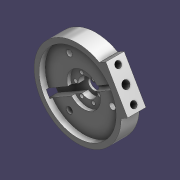
# Autodesk Inventor part: AA046
Saved by Autodesk Inventor 2017 SP1 (Build 210196100, 196)
## iProperties
Created: 2018-01-29
Part Number: AA046
Material: ABS Plastic
Document SubType Name: Modeling
Designer: Zach
Density: 1.06 g/cm^3
Appearance: CR White
Author: Zach
Autodesk Inventor part; units mm, degrees
ref_plane "YZ Plane" through (0, 0, 0) normal (1, 0, 0) x (0, 1, 0)
ref_plane "XZ Plane" through (0, 0, 0) normal (0, 1, 0) x (-1, 0, 0)
ref_plane "XY Plane" through (0, 0, 0) normal (0, 0, 1) x (1, 0, 0)
sketch "Sketch1" plane through (0, 0, 0) normal (0, 0, 1) x (1, 0, 0)
  circle A0 centre (0, 0) radius 35
  circle A1 centre (0, 0) radius 4.5
  dimension "d0" = 70
  dimension "d1" = 9
  constraints: 2 centre point, 2 coincident
  measures "d0" diameter of A0
  measures "d1" diameter of A1
extrude "Extrusion1" add sketch "Sketch1" along normal blind 14.75
sketch "Sketch2" plane through (0, 0, 14.75) normal (0, 0, 1) x (1, 0, 0)
  circle A0 centre (0, 0) radius 13.5
  dimension "d4" = 27
  constraints: 1 centre point, 1 coincident
  measures "d4" diameter of A0
extrude "Extrusion2" cut sketch "Sketch2" against normal blind 8
sketch "Sketch3" plane through (0, 0, 6.75) normal (0, 0, 1) x (1, 0, 0)
  circle A0 centre (0, 0) radius 7.5
  dimension "d7" = 15
  constraints: 1 centre point, 1 coincident
  measures "d7" diameter of A0
extrude "Extrusion3" cut sketch "Sketch3" against normal blind 5
sketch "Sketch4" plane through (0, 0, 6.75) normal (0, 0, 1) x (1, 0, 0)
  circle A0 centre (9.525, 0) radius 1.5
  circle A1 centre (4.7625, 8.2489) radius 1.5
  circle A2 centre (-4.7625, 8.2489) radius 1.5
  circle A3 centre (-9.525, 0) radius 1.5
  circle A4 centre (-4.7625, -8.2489) radius 1.5
  circle A5 centre (4.7625, -8.2489) radius 1.5
  point P0 (0, 0)
  dimension "d10" = 3
  dimension "d11" = 9.525
  dimension "d14" = 360
  constraints: 6 centre point, 1 horizontal alignment, 13 other
  measures "d10" diameter of A0
  measures "d11" distance of A0.centre point (0, 0)
extrude "Extrusion4" cut sketch "Sketch4" against normal through all
sketch "Sketch5" plane through (0, 0, 14.75) normal (0, 0, 1) x (1, 0, 0)
  circle A0 centre (23, 0) radius 2.5
  circle A1 centre (-11.5, 19.9186) radius 2.5
  circle A2 centre (-11.5, -19.9186) radius 2.5
  point P0 (0, 0)
  dimension "d18" = 5
  dimension "d19" = 23
  dimension "d22" = 360
  constraints: 3 centre point, 1 horizontal alignment, 7 other
  measures "d18" diameter of A0
  measures "d19" distance of A0.centre point (0, 0)
extrude "Extrusion5" cut sketch "Sketch5" against normal through all
sketch "Sketch6" plane through (0, 0, 14.75) normal (0, 0, 1) x (1, 0, 0)
  circle A0 centre (23, 0) radius 2.5 projected
  circle A1 centre (23, 0) radius 6.5
  circle A2 centre (11.5, 19.9186) radius 6.5
  circle A3 centre (-11.5, 19.9186) radius 6.5
  circle A4 centre (-23, 0) radius 6.5
  circle A5 centre (-11.5, -19.9186) radius 6.5
  circle A6 centre (11.5, -19.9186) radius 6.5
  point P0 (0, 0)
  dimension "d26" = 13
  dimension "d29" = 360
  constraints: 6 centre point, 1 coincident, 13 other
  measures "d26" diameter of A1
extrude "Extrusion6" cut sketch "Sketch6" against normal blind 5 contours A0 | A1 | A3 | A5
sketch "Sketch7" plane through (0, 0, 14.75) normal (0, 0, 1) x (1, 0, 0)
  line L0 (17.5, 30.3109) -> (22.6962, 33.3109)
  line L1 (22.6962, 33.3109) -> (40.1962, 3)
  line L2 (40.1962, 3) -> (35, 0)
  line L3 (35, 0) -> (17.5, 30.3109)
  circle A0 centre (0, 0) radius 35 construction
  line L4 (0, 0) -> (26.25, 15.1554)
  circle A1 centre (23, 0) radius 2.5 construction
  line L5 (0, 0) -> (23, 0)
  dimension "d33" = 6
  dimension "d34" = 35
  dimension "d43" = 30
  constraints: 12 end point, 2 parallel, 2 point on circle, 1 horizontal, 1 midpoint, 1 perpendicular
  measures "d33" distance of L0.start L0.end
  measures "d34" distance of L0.end L1.end
  measures "d43" angle of L5 L4
extrude "Extrusion7" add sketch "Sketch7" against normal blind 14.75
sketch "Sketch8" plane through (40.1962, 3, 14.75) normal (0.8660254, 0.5, 0) x (0, 0, -1)
  circle A0 centre (7.375, 30) radius 2.5
  circle A1 centre (7.375, 5) radius 2.5
  line L0 (7.375, 30) -> (7.375, 5) construction
  line L1 (14.75, 35) -> (14.75, 0) projected
  line L2 (0, 35) -> (14.75, 35) projected
  point P0 (14.75, 17.5)
  point P1 (14.75, 17.5)
  point P2 (7.375, 17.5)
  point P3 (7.375, 35)
  dimension "d37" = 5
  dimension "d38" = 5
  dimension "d39" = 25
  constraints: 3 midpoint, 2 centre point, 2 end point, 1 horizontal alignment, 1 vertical, 1 vertical alignment
  measures "d37" diameter of A0
  measures "d38" diameter of A1
  measures "d39" distance of L0.start L0.end
extrude "Extrusion8" cut sketch "Sketch8" against normal blind 10
sketch "Sketch9" plane through (40.1962, 3, 14.75) normal (0.8660254, 0.5, 0) x (0, 0, -1)
  circle A0 centre (7.375, 17.5) radius 3
  line L0 (14.75, 35) -> (14.75, 0) projected
  circle A1 centre (7.375, 30) radius 2.5 construction
  point P0 (14.75, 17.5)
  point P1 (14.75, 17.5)
  dimension "d42" = 6
  constraints: 1 centre point, 1 horizontal alignment, 1 midpoint, 1 vertical alignment
  measures "d42" diameter of A0
extrude "Extrusion9" cut sketch "Sketch9" against normal through all
ref_plane "Work Plane1" through (8.75, -15.1554, 14.75) normal (0.8660254, 0.5, 0) x (0, 0, -1)
sketch "Sketch11" plane through (8.75, -15.1554, 14.75) normal (0.8660254, 0.5, 0) x (0, 0, -1)
  line L0 (13, 22) -> (13, 13) projected
  line L1 (13, 10) -> (13, 25) projected
  line L2 (0, 35) -> (0, 0) projected
  line L3 (0, 35) -> (0, 0) projected
  line L4 (0, -0.5) -> (0, 12.5) projected
  line L5 (0, 34) -> (0, 47) projected
  line L6 (0, -0.5) -> (0, 12.5) projected
  line L7 (0, 4) -> (0, 31) projected
  line L8 (13, 10) -> (13, 25) projected
  line L9 (13, 20.5) -> (3, 20.5)
  line L10 (3, 20.5) -> (3, 14.5)
  line L11 (3, 14.5) -> (13, 14.5)
  line L12 (13, 14.5) -> (13, 20.5)
  point P0 (14.75, 17.5)
  point P1 (0, 22.5)
  point P2 (0, 35.5)
  point P3 (0, 22.5)
  point P4 (0, 35.5)
  point P5 (0, -12)
  point P6 (0, 1)
  dimension "d47" = 3
  constraints: 8 end point, 2 horizontal, 2 perpendicular, 2 point on line, 1 vertical alignment
  measures "d47" distance between parallel lines of L7 L10
extrude "Extrusion10" cut sketch "Sketch11" against normal through all
sketch "Sketch12" plane through (0, 0, 14.75) normal (0, 0, 1) x (1, 0, 0)
  arc A0 (17.5, 30.3109) -> (35, 0) centre (0, 0) ccw projected
  circle A1 centre (0, 0) radius 35
  circle A2 centre (0, 0) radius 31
  dimension "d50" = 4
  constraints: 1 centre point, 1 coincident, 1 horizontal alignment, 2 other
extrude "Extrusion11" cut sketch "Sketch12" against normal blind 5 contours A2
body "Solid1"
